007 (Autodesk Fusion 360 design; units mm, degrees)
Autodesk Fusion 360 part; units mm, degrees
sketch "Esquisse1" plane through (0, 0, 0) normal (0, 0, 1) x (1, 0, 0)
  line L0 (-52.5, 35) -> (52.5, 35)
  line L1 (52.5, 35) -> (52.5, -35)
  line L2 (-52.5, -35) -> (-52.5, 35)
  line L3 (0, 1.75) -> (0, 22.5)
  line L4 (1.75, 0) -> (22.5, 0)
  line L5 (-23.5, -35) -> (-23.5, -87)
  line L6 (-23.5, -87) -> (23.5, -87)
  line L7 (23.5, -87) -> (23.5, -35)
  line L8 (52.5, -35) -> (23.5, -35)
  line L9 (-23.5, -35) -> (-52.5, -35)
  dimension "d1" = 105
  dimension "d2" = 70
  dimension "d25" = 52
  dimension "d26" = 47
  constraint horizontal L0
  constraint vertical L1
  constraint horizontal L8
  constraint vertical L2
  constraint symmetric L1 L2 L3
  constraint coincident L5.start L8
  constraint perpendicular L5 L8
  constraint perpendicular L5 L6
  constraint perpendicular L7 L8
  constraint collinear L8 L9
  measures "d1" distance of L0.start L0.end
  measures "d2" distance of L0.start L2.start
  measures "d25" distance of L5.start L5.end
  measures "d26" distance of L5.end L6.end
extrude "Extrusion1" add sketch "Esquisse1" against normal blind 20
sketch "Esquisse3" plane through (0, 0, -20) normal (0, 0, -1) x (1, 0, 0)
  line L0 (-23.5, 35) -> (-52.5, 35)
  line L1 (-52.5, 35) -> (-52.5, -35)
  line L2 (-52.5, -35) -> (52.5, -35)
  line L3 (52.5, -35) -> (52.5, 35)
  line L4 (0, -1.75) -> (0, -22.5)
  line L5 (23.5, 87) -> (-23.5, 87)
  line L6 (-23.5, 87) -> (-23.5, 35)
  line L7 (52.5, 35) -> (23.5, 35)
  line L8 (23.5, 35) -> (23.5, 87)
  point P0 (-47, 28)
  point P1 (-23, 28)
  point P2 (-47, 10.2)
  point P3 (-23, 10.2)
  dimension "d7" = 24
  dimension "d8" = -17.8
  dimension "d16" = 47
  measures "d16" distance of P0 L4
hole "Perçage1" at (-47, -28, -20) at (-23, -28, -20) at (-23, -10.2, -20) at (-47, -10.2, -20) direction (0, 0, 1) diameter 5 depth 50 tip angle 118 counterbore diameter 8 counterbore depth 5
mirror "Symétrie miroir1" about plane through (0, 0, 0) normal (1, 0, 0) of "Perçage1"
mirror "Symétrie miroir2" about plane through (0, 0, 0) normal (0, 1, 0) of "Perçage1", "Symétrie miroir1"
sketch "Esquisse4" plane through (0, 0, -20) normal (0, 0, -1) x (1, 0, 0)
  line L0 (-23.5, 35) -> (-52.5, 35)
  line L1 (-52.5, 35) -> (-52.5, -35)
  line L2 (-52.5, -35) -> (52.5, -35)
  line L3 (52.5, -35) -> (52.5, 35)
  circle A0 centre (-40, 0) radius 4.075
  line L4 (23.5, 87) -> (-23.5, 87)
  line L5 (-23.5, 87) -> (-23.5, 35)
  line L6 (52.5, 35) -> (23.5, 35)
  line L7 (23.5, 35) -> (23.5, 87)
  circle A1 centre (23, -10.2) radius 4
  circle A2 centre (47, -28) radius 4
  circle A3 centre (23, -28) radius 4
  circle A4 centre (47, -10.2) radius 4
  circle A5 centre (-23, -10.2) radius 4
  circle A6 centre (-47, -28) radius 4
  circle A7 centre (-23, -28) radius 4
  circle A8 centre (-47, -10.2) radius 4
  circle A9 centre (23, 10.2) radius 4
  circle A10 centre (47, 28) radius 4
  circle A11 centre (23, 28) radius 4
  circle A12 centre (47, 10.2) radius 4
  circle A13 centre (-23, 10.2) radius 4
  circle A14 centre (-47, 28) radius 4
  circle A15 centre (-23, 28) radius 4
  circle A16 centre (-47, 10.2) radius 4
  dimension "d17" = 8.15
  dimension "d18" = 40
  measures "d17" diameter of A0
  measures "d18" distance of origin A0.centre
extrude "Extrusion2" cut sketch "Esquisse4" against normal blind 15 contours A0
mirror "Symétrie miroir3" about plane through (0, 0, 0) normal (1, 0, 0) of "Extrusion2"
sketch "Esquisse6" plane through (0, 0, -20) normal (0, 0, -1) x (1, 0, 0)
  circle A0 centre (40, 0) radius 4.075
  circle A1 centre (-40, 0) radius 4.075
  line L0 (23.5, 87) -> (-23.5, 87)
  line L1 (-23.5, 87) -> (-23.5, 35)
  line L2 (-23.5, 35) -> (-52.5, 35)
  line L3 (-52.5, 35) -> (-52.5, -35)
  line L4 (-52.5, -35) -> (52.5, -35)
  line L5 (52.5, -35) -> (52.5, 35)
  line L6 (52.5, 35) -> (23.5, 35)
  line L7 (23.5, 35) -> (23.5, 87)
  line L8 (-21.1, 77) -> (21.1, 77)
  line L9 (21.1, 77) -> (21.1, 34.8)
  line L10 (21.1, 34.8) -> (-21.1, 34.8)
  line L11 (-21.1, 34.8) -> (-21.1, 77)
  line L12 (0, -1.75) -> (0, -22.5)
  circle A2 centre (23, -10.2) radius 4
  circle A3 centre (47, -28) radius 4
  circle A4 centre (23, -28) radius 4
  circle A5 centre (47, -10.2) radius 4
  circle A6 centre (-23, -10.2) radius 4
  circle A7 centre (-47, -28) radius 4
  circle A8 centre (-23, -28) radius 4
  circle A9 centre (-47, -10.2) radius 4
  circle A10 centre (23, 10.2) radius 4
  circle A11 centre (47, 28) radius 4
  circle A12 centre (23, 28) radius 4
  circle A13 centre (47, 10.2) radius 4
  circle A14 centre (-23, 10.2) radius 4
  circle A15 centre (-47, 28) radius 4
  circle A16 centre (-23, 28) radius 4
  circle A17 centre (-47, 10.2) radius 4
  dimension "d27" = 42.2
  dimension "d28" = 42.2
  dimension "d29" = 10
  constraint horizontal L8
  constraint vertical L9
  constraint horizontal L10
  constraint vertical L11
  constraint symmetric L9 L11 L12
  measures "d27" distance of L8.start L8.end
  measures "d28" distance of L8.start L10.end
  measures "d29" distance of L0 L8
extrude "Extrusion3" cut sketch "Esquisse6" against normal blind 12 contours L8 L9 L10 L11
sketch "Esquisse7" plane through (0, 0, -8) normal (0, 0, -1) x (1, 0, 0)
  line L0 (-21.1, 34.8) -> (21.1, 34.8)
  line L1 (21.1, 34.8) -> (21.1, 77)
  line L2 (21.1, 77) -> (-21.1, 77)
  line L3 (-21.1, 77) -> (-21.1, 34.8)
  circle A0 centre (0, 55.9) radius 11.1
  line L4 (-21.1, 77) -> (21.1, 77)
  line L5 (0, -1.75) -> (0, -22.5)
  dimension "d32" = 22.2
  dimension "d33" = 21.1
  constraint coincident A0.centre L5
  measures "d32" diameter of A0
  measures "d33" distance of A0.centre L4
extrude "Extrusion4" cut sketch "Esquisse7" against normal blind 2.5 contours A0
sketch "Esquisse8" plane through (0, 0, -5.5) normal (0, 0, -1) x (1, 0, 0)
  circle A0 centre (0, 55.9) radius 11.1
  circle A1 centre (0, 55.9) radius 4
  dimension "d36" = 8
  constraint concentric A0 A1
  measures "d36" diameter of A1
extrude "Extrusion5" cut sketch "Esquisse8" against normal blind 9 contours A1
sketch "Esquisse9" plane through (0, 0, -20) normal (0, 0, -1) x (1, 0, 0)
  line L0 (21.1, 77) -> (21.1, 34.8)
  line L1 (21.1, 34.8) -> (-21.1, 34.8)
  line L2 (-21.1, 34.8) -> (-21.1, 77)
  line L3 (-21.1, 77) -> (21.1, 77)
  circle A0 centre (40, 0) radius 4.075
  circle A1 centre (-40, 0) radius 4.075
  line L4 (23.5, 87) -> (-23.5, 87)
  line L5 (-23.5, 87) -> (-23.5, 35)
  line L6 (-23.5, 35) -> (-52.5, 35)
  line L7 (-52.5, 35) -> (-52.5, -35)
  line L8 (-52.5, -35) -> (52.5, -35)
  line L9 (52.5, -35) -> (52.5, 35)
  line L10 (52.5, 35) -> (23.5, 35)
  line L11 (23.5, 35) -> (23.5, 87)
  circle A2 centre (0, 0) radius 11.15
  circle A3 centre (23, -10.2) radius 4
  circle A4 centre (47, -28) radius 4
  circle A5 centre (23, -28) radius 4
  circle A6 centre (47, -10.2) radius 4
  circle A7 centre (-23, -10.2) radius 4
  circle A8 centre (-47, -28) radius 4
  circle A9 centre (-23, -28) radius 4
  circle A10 centre (-47, -10.2) radius 4
  circle A11 centre (23, 10.2) radius 4
  circle A12 centre (47, 28) radius 4
  circle A13 centre (23, 28) radius 4
  circle A14 centre (47, 10.2) radius 4
  circle A15 centre (-23, 10.2) radius 4
  circle A16 centre (-47, 28) radius 4
  circle A17 centre (-23, 28) radius 4
  circle A18 centre (-47, 10.2) radius 4
  dimension "d39" = 22.3
  constraint coincident A2.centre origin
  measures "d39" diameter of A2
extrude "Extrusion6" cut sketch "Esquisse9" against normal blind 8 contours A2
sketch "Esquisse10" plane through (0, 0, 0) normal (0, 0, 1) x (-1, 0, 0)
  circle A0 centre (-23, -10.2) radius 2.5
  circle A1 centre (-47, -28) radius 2.5
  circle A2 centre (-23, -28) radius 2.5
  circle A3 centre (-47, -10.2) radius 2.5
  circle A4 centre (23, -10.2) radius 2.5
  circle A5 centre (47, -28) radius 2.5
  circle A6 centre (23, -28) radius 2.5
  circle A7 centre (47, -10.2) radius 2.5
  circle A8 centre (-23, 10.2) radius 2.5
  circle A9 centre (-47, 28) radius 2.5
  circle A10 centre (-23, 28) radius 2.5
  circle A11 centre (-47, 10.2) radius 2.5
  circle A12 centre (23, 10.2) radius 2.5
  circle A13 centre (47, 28) radius 2.5
  circle A14 centre (23, 28) radius 2.5
  circle A15 centre (47, 10.2) radius 2.5
  line L0 (23.5, 87) -> (-23.5, 87)
  line L1 (-23.5, 87) -> (-23.5, 35)
  line L2 (-23.5, 35) -> (-52.5, 35)
  line L3 (-52.5, 35) -> (-52.5, -35)
  line L4 (-52.5, -35) -> (52.5, -35)
  line L5 (52.5, -35) -> (52.5, 35)
  line L6 (52.5, 35) -> (23.5, 35)
  line L7 (23.5, 35) -> (23.5, 87)
  circle A16 centre (0, 0) radius 11.15
  circle A17 centre (0, 55.9) radius 4
  dimension "d42" = 22.3
  constraint coincident A16.centre origin
  measures "d42" diameter of A16
extrude "Extrusion7" cut sketch "Esquisse10" against normal blind 8 contours A16
sketch "Esquisse11" plane through (0, 0, -12) normal (0, 0, -1) x (1, 0, 0)
  circle A0 centre (0, 0) radius 11.15
  circle A1 centre (0, 0) radius 4.5
  dimension "d45" = 9
  constraint coincident A0.centre A1.centre
  measures "d45" diameter of A1
extrude "Extrusion8" cut sketch "Esquisse11" against normal blind 15 contours A1
sketch "Esquisse12" plane through (0, 0, -8) normal (0, 0, -1) x (1, 0, 0)
  circle A0 centre (0, 55.9) radius 11.1
  line L0 (-21.1, 34.8) -> (21.1, 34.8)
  line L1 (21.1, 34.8) -> (21.1, 77)
  line L2 (21.1, 77) -> (-21.1, 77)
  line L3 (-21.1, 77) -> (-21.1, 34.8)
  point P0 (-15.5, 71.4)
  point P1 (15.5, 71.4)
  point P2 (-15.5, 40.4)
  point P3 (15.5, 40.4)
  dimension "d48" = 15.5
  dimension "d49" = 15.5
  dimension "d52" = 31
  dimension "d53" = -31
  measures "d48" horizontal distance of A0.centre P0
  measures "d49" vertical distance of A0.centre P0
hole "Perçage2" at (-15.5, -71.4, -8) at (15.5, -71.4, -8) at (15.5, -40.4, -8) at (-15.5, -40.4, -8) direction (0, 0, 1) diameter 4 depth 50 tip angle 118
sketch "Esquisse13" plane through (0, 0, 0) normal (0, 0, 1) x (-1, 0, 0)
  circle A0 centre (-15.5, 40.4) radius 2
  circle A1 centre (15.5, 71.4) radius 2
  circle A2 centre (-15.5, 71.4) radius 2
  circle A3 centre (15.5, 40.4) radius 2
  circle A4 centre (0, 0) radius 11.15
  circle A5 centre (0, 55.9) radius 4
  circle A6 centre (-23, -10.2) radius 2.5
  circle A7 centre (-47, -28) radius 2.5
  circle A8 centre (-23, -28) radius 2.5
  circle A9 centre (-47, -10.2) radius 2.5
  circle A10 centre (23, -10.2) radius 2.5
  circle A11 centre (47, -28) radius 2.5
  circle A12 centre (23, -28) radius 2.5
  circle A13 centre (47, -10.2) radius 2.5
  circle A14 centre (-23, 10.2) radius 2.5
  circle A15 centre (-47, 28) radius 2.5
  circle A16 centre (-23, 28) radius 2.5
  circle A17 centre (-47, 10.2) radius 2.5
  circle A18 centre (23, 10.2) radius 2.5
  circle A19 centre (47, 28) radius 2.5
  circle A20 centre (23, 28) radius 2.5
  circle A21 centre (47, 10.2) radius 2.5
  line L0 (23.5, 87) -> (-23.5, 87)
  line L1 (-23.5, 87) -> (-23.5, 35)
  line L2 (-23.5, 35) -> (-52.5, 35)
  line L3 (-52.5, 35) -> (-52.5, -35)
  line L4 (-52.5, -35) -> (52.5, -35)
  line L5 (52.5, -35) -> (52.5, 35)
  line L6 (52.5, 35) -> (23.5, 35)
  line L7 (23.5, 35) -> (23.5, 87)
  point P0 (11, -30)
  dimension "d57" = 30
  dimension "d58" = 11
  measures "d57" vertical distance of A4.centre P0
  measures "d58" horizontal distance of A4.centre P0
hole "Perçage3" at (-11, 30, 0) direction (0, 0, -1) diameter 4.5 depth 50 tip angle 118
mirror "Symétrie miroir4" about plane through (0, 0, 0) normal (1, 0, 0) of "Perçage3"
pattern_linear "Réseau R1" count 2 spacing 110.5 along (0, -1, 0) of "Perçage3", "Symétrie miroir4"
sketch "Esquisse14" plane through (0, 0, 0) normal (0, 0, 1) x (-1, 0, 0)
  circle A0 centre (-11, 80.5) radius 2.25
  circle A1 centre (11, 80.5) radius 2.25
  circle A2 centre (-11, -30) radius 2.25
  circle A3 centre (11, -30) radius 2.25
  circle A4 centre (-15.5, 40.4) radius 2
  circle A5 centre (15.5, 71.4) radius 2
  circle A6 centre (-15.5, 71.4) radius 2
  circle A7 centre (15.5, 40.4) radius 2
  circle A8 centre (0, 0) radius 11.15
  circle A9 centre (0, 55.9) radius 4
  circle A10 centre (-23, -10.2) radius 2.5
  circle A11 centre (-47, -28) radius 2.5
  circle A12 centre (-23, -28) radius 2.5
  circle A13 centre (-47, -10.2) radius 2.5
  circle A14 centre (23, -10.2) radius 2.5
  circle A15 centre (47, -28) radius 2.5
  circle A16 centre (23, -28) radius 2.5
  circle A17 centre (47, -10.2) radius 2.5
  circle A18 centre (-23, 10.2) radius 2.5
  circle A19 centre (-47, 28) radius 2.5
  circle A20 centre (-23, 28) radius 2.5
  circle A21 centre (-47, 10.2) radius 2.5
  circle A22 centre (23, 10.2) radius 2.5
  circle A23 centre (47, 28) radius 2.5
  circle A24 centre (23, 28) radius 2.5
  circle A25 centre (47, 10.2) radius 2.5
  line L0 (23.5, 87) -> (-23.5, 87)
  line L1 (-23.5, 87) -> (-23.5, 35)
  line L2 (-23.5, 35) -> (-52.5, 35)
  line L3 (-52.5, 35) -> (-52.5, -35)
  line L4 (-52.5, -35) -> (52.5, -35)
  line L5 (52.5, -35) -> (52.5, 35)
  line L6 (52.5, 35) -> (23.5, 35)
  line L7 (23.5, 35) -> (23.5, 87)
  circle A26 centre (0, -20) radius 1.3
  line L8 (-20, 0) -> (-2.5, 0)
  dimension "d70" = 2.6
  dimension "d71" = 20
  measures "d70" diameter of A26
  measures "d71" distance of A26.centre L8
extrude "Extrusion9" cut sketch "Esquisse14" against normal blind 24 contours A26
mirror "Symétrie miroir5" about plane through (0, 0, 0) normal (0, 1, 0) of "Extrusion9"
fillet "Congé1" radius 5 8 edges at (-52.5, 35, -10) (52.5, 35, -10) (52.5, -35, -10) (23.5, -87, -10) (-23.5, -87, -10) (-23.5, -35, -10) (23.5, -35, -10) (-52.5, -35, -10)
equation "d16 = ( ( 70 / 2 ) * 1 mm ) + 12 mm"
equation "d32 = ( 11.10 * 2 ) * 1 mm"
equation "d33 = ( 42.2 / 2 ) * 1 mm"
equation "d48 = ( 31 / 2 ) * 1 mm"
equation "d49 = ( 31 / 2 ) * 1 mm"
